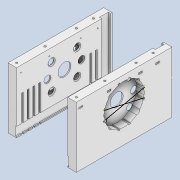
# Autodesk Inventor part: corpus_90x90x140mm_side_walls_LED_Irradiation_Firesting_ports
Saved by Autodesk Inventor 2021 (Build 250183000, 183)
## iProperties
Created: 2020-02-19
Part Number: corpus_90x90x140mm_side_walls_LED_Irradiation_Firesting_ports
Material: Acetalharz, Weiß
Document SubType Name: Modeling
Designer: Daniel
Density: 1.425 g/cm^3
Appearance: Glatt - Weiß
Author: Daniel
Autodesk Inventor part; units mm, degrees
(part 1 of 2)
ref_plane "YZ Plane" through (0, 0, 0) normal (1, 0, 0) x (0, 1, 0)
ref_plane "XZ Plane" through (0, 0, 0) normal (0, 1, 0) x (-1, 0, 0)
sketch "Skizze1" plane through (0, 0, 0) normal (0, 0, 1) x (1, 0, 0)
  line L0 (-60, 61) -> (60, 61)
  line L1 (60, 61) -> (60, -61)
  line L2 (60, -61) -> (-60, -61)
  line L3 (-60, -61) -> (-60, 61)
  line L4 (-60, 61) -> (60, -61) construction
  line L5 (60, 61) -> (-60, -61) construction
  line L6 (-45, 45.75) -> (45, 45.75)
  line L7 (45, 45.75) -> (45, -45.75)
  line L8 (45, -45.75) -> (-45, -45.75)
  line L9 (-45, -45.75) -> (-45, 45.75)
  line L10 (-45, 45.75) -> (45, -45.75) construction
  line L11 (45, 45.75) -> (-45, -45.75) construction
  line L12 (-45, -45.75) -> (-45, -61)
  line L13 (-45, -61) -> (45, -61)
  line L14 (45, -61) -> (45, -45.75)
  line L15 (45, -45.75) -> (-45, -45.75)
  line L16 (45, -43.5) -> (47, -43.5)
  line L17 (47, -43.5) -> (47, -59)
  line L18 (47, -59) -> (45, -59)
  line L19 (45, -59) -> (45, -43.5)
  line L20 (-45, -43.5) -> (-47, -43.5)
  line L21 (-47, -43.5) -> (-47, -59)
  line L22 (-47, -59) -> (-45, -59)
  line L23 (-45, -59) -> (-45, -43.5)
  point P0 (0, 0)
  dimension "d0" = 120
  dimension "d1" = 122
  dimension "d2" = 90
  dimension "d3" = 15.5
  dimension "d4" = 15.5
  dimension "d5" = 2
  dimension "d6" = 2
  dimension "d7" = 2
  dimension "d93" = 94
  dimension "d96" = 2
  constraints: 48 end point, 10 parallel, 9 point on line, 6 perpendicular, 4 midpoint, 2 horizontal
  measures "d0" distance of L0.start L0.end
  measures "d1" distance of L0.end L1.end
  measures "d2" distance of L6.start L6.end
  measures "d3" distance of L16.end L17.end
  measures "d4" distance of L20.end L21.end
  measures "d5" distance of L17.end L18.end
  measures "d6" distance of L21.end L22.end
  measures "d7" distance between parallel lines of L2 L18
  measures "d93" distance between parallel lines of L17 L21
  measures "d96" distance between parallel lines of L2 L22
extrude "Extrusion1" add sketch "Skizze1" along normal blind 168 contours L0 L1 L2 L14 L18 L17 L16 L7 L6 L9 L20 L21 L22 L12 L3
sketch "Skizze2" plane through (-60, -61, 0) normal (0, -1, 0) x (1, 0, 0)
  line L0 (10.8, 18.5) -> (109.2, 18.5)
  line L1 (109.2, 18.5) -> (109.2, 3)
  line L2 (109.2, 3) -> (10.8, 3)
  line L3 (10.8, 3) -> (10.8, 18.5)
  line L4 (10.8, 18.5) -> (109.2, 3) construction
  line L5 (109.2, 18.5) -> (10.8, 3) construction
  line L6 (105, 0) -> (120, 0) projected
  point P0 (60, 0)
  point P1 (60, 10.75)
  dimension "d10" = 10.75
  dimension "d11" = 98.4
  dimension "d12" = 15.5
  constraints: 12 end point, 2 midpoint, 2 parallel, 1 horizontal, 1 perpendicular
  measures "d10" distance of point (60, 0) point (60, 10.75)
  measures "d11" distance of L0.start L0.end
  measures "d12" distance of L0.end L1.end
extrude "Extrusion2" cut sketch "Skizze2" against normal blind 112
sketch "Skizze3" plane through (-45, 45.75, 168) normal (0, -1, 0) x (1, 0, 0)
  line L0 (-15, -168) -> (-15, 0) projected
  line L1 (105, -168) -> (105, 0) projected
  line L2 (-15, 0) -> (105, 0)
  line L3 (105, 0) -> (105, -120)
  line L4 (105, -120) -> (-15, -120)
  line L5 (-15, -120) -> (-15, 0)
  line L6 (105, 0) -> (-15, 0) construction
  line L7 (-15, 0) -> (105, -120) construction
  line L8 (105, -168) -> (105, 0) construction
  line L9 (105, 0) -> (-15, -120) construction
  circle A0 centre (45, -60) radius 45
  point P0 (45, -168)
  dimension "d16" = 120
  dimension "d17" = 90
  constraints: 12 end point, 2 parallel, 1 centre point, 1 coincident, 1 horizontal, 1 midpoint, 1 perpendicular, 1 point on line
  measures "d16" distance from line of L4 L1.end
  measures "d17" diameter of A0
extrude "Extrusion3" cut sketch "Skizze3" against normal up to surface (15.25 mm away) contours A0
sketch "Skizze4" plane through (-60, 61, 0) normal (0, 1, 0) x (1, 0, 0)
  arc A0 (105, -108) -> (15, -108) centre (60, -108) ccw projected
  circle A1 centre (60, -108) radius 45
  line L0 (120, 0) -> (120, -168) construction
  line L1 (0, 0) -> (0, -168) construction
  line L2 (120, -168) -> (0, -168) construction
  line L3 (0, -168) -> (0, -48) construction
  line L4 (0, -48) -> (120, -48) construction
  line L5 (120, -48) -> (120, -168) construction
  line L6 (0, -168) -> (120, -48) construction
  line L7 (120, -168) -> (0, -48) construction
  line L8 (24.9924, -114.4218) -> (23.5782, -113.0076)
  line L9 (23.5782, -113.0076) -> (95.0076, -41.5782)
  line L10 (95.0076, -41.5782) -> (96.4218, -42.9924)
  line L11 (96.4218, -42.9924) -> (24.9924, -114.4218)
  line L12 (59, -57.4918) -> (61, -158.5082) construction
  line L13 (61, -57.4918) -> (59, -158.5082) construction
  line L14 (23.1391, -39.7249) -> (98.2751, -114.8609)
  line L15 (98.2751, -114.8609) -> (96.8609, -116.2751)
  line L16 (96.8609, -116.2751) -> (21.7249, -41.1391)
  line L17 (21.7249, -41.1391) -> (23.1391, -39.7249)
  line L18 (113.1292, -109) -> (6.8708, -107) construction
  line L19 (6.8708, -109) -> (113.1292, -107) construction
  line L20 (30.2102, -32.6538) -> (105.3462, -107.7898)
  line L21 (103.932, -109.2041) -> (28.7959, -34.068)
  line L22 (28.7959, -34.068) -> (30.2102, -32.6538)
  line L23 (105.3462, -107.7898) -> (103.932, -109.2041)
  line L24 (37.2812, -25.5827) -> (112.4173, -100.7188)
  line L25 (111.003, -102.133) -> (35.867, -26.997)
  line L26 (35.867, -26.997) -> (37.2812, -25.5827)
  line L27 (112.4173, -100.7188) -> (111.003, -102.133)
  line L28 (44.3523, -18.5117) -> (119.4883, -93.6477)
  line L29 (118.0741, -95.0619) -> (42.9381, -19.9259)
  line L30 (42.9381, -19.9259) -> (44.3523, -18.5117)
  line L31 (119.4883, -93.6477) -> (118.0741, -95.0619)
  line L32 (51.4234, -11.4406) -> (126.5594, -86.5766)
  line L33 (125.1452, -87.9909) -> (50.0091, -12.8548)
  line L34 (50.0091, -12.8548) -> (51.4234, -11.4406)
  line L35 (126.5594, -86.5766) -> (125.1452, -87.9909)
  line L36 (16.068, -46.7959) -> (91.2041, -121.932)
  line L37 (89.7898, -123.3462) -> (14.6538, -48.2102)
  line L38 (14.6538, -48.2102) -> (16.068, -46.7959)
  line L39 (91.2041, -121.932) -> (89.7898, -123.3462)
  line L40 (23.1391, -39.7249) -> (98.2751, -114.8609)
  line L41 (96.8609, -116.2751) -> (21.7249, -41.1391)
  line L42 (21.7249, -41.1391) -> (23.1391, -39.7249)
  line L43 (98.2751, -114.8609) -> (96.8609, -116.2751)
  line L44 (30.2102, -32.6538) -> (105.3462, -107.7898)
  line L45 (103.932, -109.2041) -> (28.7959, -34.068)
  line L46 (28.7959, -34.068) -> (30.2102, -32.6538)
  line L47 (105.3462, -107.7898) -> (103.932, -109.2041)
  line L48 (37.2812, -25.5827) -> (112.4173, -100.7188)
  line L49 (111.003, -102.133) -> (35.867, -26.997)
  line L50 (35.867, -26.997) -> (37.2812, -25.5827)
  line L51 (112.4173, -100.7188) -> (111.003, -102.133)
  line L52 (44.3523, -18.5117) -> (119.4883, -93.6477)
  line L53 (118.0741, -95.0619) -> (42.9381, -19.9259)
  line L54 (42.9381, -19.9259) -> (44.3523, -18.5117)
  line L55 (119.4883, -93.6477) -> (118.0741, -95.0619)
  line L56 (8.997, -53.867) -> (84.133, -129.003)
  line L57 (82.7188, -130.4173) -> (7.5827, -55.2812)
  line L58 (7.5827, -55.2812) -> (8.997, -53.867)
  line L59 (84.133, -129.003) -> (82.7188, -130.4173)
  line L60 (16.068, -46.7959) -> (91.2041, -121.932)
  line L61 (89.7898, -123.3462) -> (14.6538, -48.2102)
  line L62 (14.6538, -48.2102) -> (16.068, -46.7959)
  line L63 (91.2041, -121.932) -> (89.7898, -123.3462)
  line L64 (23.1391, -39.7249) -> (98.2751, -114.8609)
  line L65 (96.8609, -116.2751) -> (21.7249, -41.1391)
  line L66 (21.7249, -41.1391) -> (23.1391, -39.7249)
  line L67 (98.2751, -114.8609) -> (96.8609, -116.2751)
  line L68 (30.2102, -32.6538) -> (105.3462, -107.7898)
  line L69 (103.932, -109.2041) -> (28.7959, -34.068)
  line L70 (28.7959, -34.068) -> (30.2102, -32.6538)
  line L71 (105.3462, -107.7898) -> (103.932, -109.2041)
  line L72 (37.2812, -25.5827) -> (112.4173, -100.7188)
  line L73 (111.003, -102.133) -> (35.867, -26.997)
  line L74 (35.867, -26.997) -> (37.2812, -25.5827)
  line L75 (112.4173, -100.7188) -> (111.003, -102.133)
  line L76 (1.9259, -60.9381) -> (77.0619, -136.0741)
  line L77 (75.6477, -137.4883) -> (0.5117, -62.3523)
  line L78 (0.5117, -62.3523) -> (1.9259, -60.9381)
  line L79 (77.0619, -136.0741) -> (75.6477, -137.4883)
  line L80 (8.997, -53.867) -> (84.133, -129.003)
  line L81 (82.7188, -130.4173) -> (7.5827, -55.2812)
  line L82 (7.5827, -55.2812) -> (8.997, -53.867)
  line L83 (84.133, -129.003) -> (82.7188, -130.4173)
  line L84 (16.068, -46.7959) -> (91.2041, -121.932)
  line L85 (89.7898, -123.3462) -> (14.6538, -48.2102)
  line L86 (14.6538, -48.2102) -> (16.068, -46.7959)
  line L87 (91.2041, -121.932) -> (89.7898, -123.3462)
  line L88 (23.1391, -39.7249) -> (98.2751, -114.8609)
  line L89 (96.8609, -116.2751) -> (21.7249, -41.1391)
  line L90 (21.7249, -41.1391) -> (23.1391, -39.7249)
  line L91 (98.2751, -114.8609) -> (96.8609, -116.2751)
  line L92 (30.2102, -32.6538) -> (105.3462, -107.7898)
  line L93 (103.932, -109.2041) -> (28.7959, -34.068)
  line L94 (28.7959, -34.068) -> (30.2102, -32.6538)
  line L95 (105.3462, -107.7898) -> (103.932, -109.2041)
  line L96 (-5.1452, -68.0091) -> (69.9909, -143.1452)
  line L97 (68.5766, -144.5594) -> (-6.5594, -69.4234)
  line L98 (-6.5594, -69.4234) -> (-5.1452, -68.0091)
  line L99 (69.9909, -143.1452) -> (68.5766, -144.5594)
  line L100 (1.9259, -60.9381) -> (77.0619, -136.0741)
  line L101 (75.6477, -137.4883) -> (0.5117, -62.3523)
  line L102 (0.5117, -62.3523) -> (1.9259, -60.9381)
  line L103 (77.0619, -136.0741) -> (75.6477, -137.4883)
  line L104 (8.997, -53.867) -> (84.133, -129.003)
  line L105 (82.7188, -130.4173) -> (7.5827, -55.2812)
  line L106 (7.5827, -55.2812) -> (8.997, -53.867)
  line L107 (84.133, -129.003) -> (82.7188, -130.4173)
  line L108 (16.068, -46.7959) -> (91.2041, -121.932)
  line L109 (89.7898, -123.3462) -> (14.6538, -48.2102)
  line L110 (14.6538, -48.2102) -> (16.068, -46.7959)
  line L111 (91.2041, -121.932) -> (89.7898, -123.3462)
  line L112 (23.1391, -39.7249) -> (98.2751, -114.8609)
  line L113 (96.8609, -116.2751) -> (21.7249, -41.1391)
  line L114 (21.7249, -41.1391) -> (23.1391, -39.7249)
  line L115 (98.2751, -114.8609) -> (96.8609, -116.2751)
  line L116 (16.5071, -105.9365) -> (87.9365, -34.5071)
  line L117 (89.3507, -35.9213) -> (17.9213, -107.3507)
  line L118 (17.9213, -107.3507) -> (16.5071, -105.9365)
  line L119 (87.9365, -34.5071) -> (89.3507, -35.9213)
  line L120 (9.4361, -98.8655) -> (80.8655, -27.4361)
  line L121 (82.2797, -28.8503) -> (10.8503, -100.2797)
  line L122 (10.8503, -100.2797) -> (9.4361, -98.8655)
  line L123 (80.8655, -27.4361) -> (82.2797, -28.8503)
  line L124 (2.365, -91.7944) -> (73.7944, -20.365)
  line L125 (75.2086, -21.7792) -> (3.7792, -93.2086)
  line L126 (3.7792, -93.2086) -> (2.365, -91.7944)
  line L127 (73.7944, -20.365) -> (75.2086, -21.7792)
  line L128 (-4.7061, -84.7233) -> (66.7233, -13.2939)
  line L129 (68.1375, -14.7081) -> (-3.2919, -86.1375)
  line L130 (-3.2919, -86.1375) -> (-4.7061, -84.7233)
  line L131 (66.7233, -13.2939) -> (68.1375, -14.7081)
  line L132 (30.6493, -120.0787) -> (102.0787, -48.6493)
  line L133 (103.4929, -50.0635) -> (32.0635, -121.4929)
  line L134 (32.0635, -121.4929) -> (30.6493, -120.0787)
  line L135 (102.0787, -48.6493) -> (103.4929, -50.0635)
  line L136 (23.5782, -113.0076) -> (95.0076, -41.5782)
  line L137 (96.4218, -42.9924) -> (24.9924, -114.4218)
  line L138 (24.9924, -114.4218) -> (23.5782, -113.0076)
  line L139 (95.0076, -41.5782) -> (96.4218, -42.9924)
  line L140 (16.5071, -105.9365) -> (87.9365, -34.5071)
  line L141 (89.3507, -35.9213) -> (17.9213, -107.3507)
  line L142 (17.9213, -107.3507) -> (16.5071, -105.9365)
  line L143 (87.9365, -34.5071) -> (89.3507, -35.9213)
  line L144 (9.4361, -98.8655) -> (80.8655, -27.4361)
  line L145 (82.2797, -28.8503) -> (10.8503, -100.2797)
  line L146 (10.8503, -100.2797) -> (9.4361, -98.8655)
  line L147 (80.8655, -27.4361) -> (82.2797, -28.8503)
  line L148 (2.365, -91.7944) -> (73.7944, -20.365)
  line L149 (75.2086, -21.7792) -> (3.7792, -93.2086)
  line L150 (3.7792, -93.2086) -> (2.365, -91.7944)
  line L151 (73.7944, -20.365) -> (75.2086, -21.7792)
  line L152 (37.7203, -127.1497) -> (109.1497, -55.7203)
  line L153 (110.5639, -57.1345) -> (39.1345, -128.5639)
  line L154 (39.1345, -128.5639) -> (37.7203, -127.1497)
  line L155 (109.1497, -55.7203) -> (110.5639, -57.1345)
  line L156 (30.6493, -120.0787) -> (102.0787, -48.6493)
  line L157 (103.4929, -50.0635) -> (32.0635, -121.4929)
  line L158 (32.0635, -121.4929) -> (30.6493, -120.0787)
  line L159 (102.0787, -48.6493) -> (103.4929, -50.0635)
  line L160 (23.5782, -113.0076) -> (95.0076, -41.5782)
  line L161 (96.4218, -42.9924) -> (24.9924, -114.4218)
  line L162 (24.9924, -114.4218) -> (23.5782, -113.0076)
  line L163 (95.0076, -41.5782) -> (96.4218, -42.9924)
  line L164 (16.5071, -105.9365) -> (87.9365, -34.5071)
  line L165 (89.3507, -35.9213) -> (17.9213, -107.3507)
  line L166 (17.9213, -107.3507) -> (16.5071, -105.9365)
  line L167 (87.9365, -34.5071) -> (89.3507, -35.9213)
  line L168 (9.4361, -98.8655) -> (80.8655, -27.4361)
  line L169 (82.2797, -28.8503) -> (10.8503, -100.2797)
  line L170 (10.8503, -100.2797) -> (9.4361, -98.8655)
  line L171 (80.8655, -27.4361) -> (82.2797, -28.8503)
  line L172 (44.7914, -134.2208) -> (116.2208, -62.7914)
  line L173 (117.635, -64.2056) -> (46.2056, -135.635)
  line L174 (46.2056, -135.635) -> (44.7914, -134.2208)
  line L175 (116.2208, -62.7914) -> (117.635, -64.2056)
  line L176 (37.7203, -127.1497) -> (109.1497, -55.7203)
  line L177 (110.5639, -57.1345) -> (39.1345, -128.5639)
  line L178 (39.1345, -128.5639) -> (37.7203, -127.1497)
  line L179 (109.1497, -55.7203) -> (110.5639, -57.1345)
  line L180 (30.6493, -120.0787) -> (102.0787, -48.6493)
  line L181 (103.4929, -50.0635) -> (32.0635, -121.4929)
  line L182 (32.0635, -121.4929) -> (30.6493, -120.0787)
  line L183 (102.0787, -48.6493) -> (103.4929, -50.0635)
  line L184 (23.5782, -113.0076) -> (95.0076, -41.5782)
  line L185 (96.4218, -42.9924) -> (24.9924, -114.4218)
  line L186 (24.9924, -114.4218) -> (23.5782, -113.0076)
  line L187 (95.0076, -41.5782) -> (96.4218, -42.9924)
  line L188 (16.5071, -105.9365) -> (87.9365, -34.5071)
  line L189 (89.3507, -35.9213) -> (17.9213, -107.3507)
  line L190 (17.9213, -107.3507) -> (16.5071, -105.9365)
  line L191 (87.9365, -34.5071) -> (89.3507, -35.9213)
  line L192 (51.8625, -141.2919) -> (123.2919, -69.8625)
  line L193 (124.7061, -71.2767) -> (53.2767, -142.7061)
  line L194 (53.2767, -142.7061) -> (51.8625, -141.2919)
  line L195 (123.2919, -69.8625) -> (124.7061, -71.2767)
  line L196 (44.7914, -134.2208) -> (116.2208, -62.7914)
  line L197 (117.635, -64.2056) -> (46.2056, -135.635)
  line L198 (46.2056, -135.635) -> (44.7914, -134.2208)
  line L199 (116.2208, -62.7914) -> (117.635, -64.2056)
  line L200 (37.7203, -127.1497) -> (109.1497, -55.7203)
  line L201 (110.5639, -57.1345) -> (39.1345, -128.5639)
  line L202 (39.1345, -128.5639) -> (37.7203, -127.1497)
  line L203 (109.1497, -55.7203) -> (110.5639, -57.1345)
  line L204 (30.6493, -120.0787) -> (102.0787, -48.6493)
  line L205 (103.4929, -50.0635) -> (32.0635, -121.4929)
  line L206 (32.0635, -121.4929) -> (30.6493, -120.0787)
  line L207 (102.0787, -48.6493) -> (103.4929, -50.0635)
  line L208 (23.5782, -113.0076) -> (95.0076, -41.5782)
  line L209 (96.4218, -42.9924) -> (24.9924, -114.4218)
  line L210 (24.9924, -114.4218) -> (23.5782, -113.0076)
  line L211 (95.0076, -41.5782) -> (96.4218, -42.9924)
  point P0 (60, 0)
  point P1 (60, -79.4142)
  point P2 (65.6569, -85.0711)
  point P3 (60, -90.7279)
  point P4 (54.3431, -85.0711)
  point P5 (58.5858, -78)
  point P6 (52.9289, -83.6569)
  point P7 (47.2721, -78)
  point P8 (52.9289, -72.3431)
  point P9 (60, -76.5858)
  point P10 (54.3431, -70.9289)
  point P11 (60, -65.2721)
  point P12 (65.6569, -70.9289)
  point P13 (61.4142, -78)
  point P14 (67.0711, -72.3431)
  point P15 (72.7279, -78)
  point P16 (67.0711, -83.6569)
  point P17 (75.5563, -63.8579)
  point P18 (81.2132, -58.201)
  point P19 (86.8701, -63.8579)
  point P20 (81.2132, -69.5147)
  point P21 (74.1421, -62.4437)
  point P22 (68.4853, -56.7868)
  point P23 (74.1421, -51.1299)
  point P24 (79.799, -56.7868)
  point P25 (88.2843, -48.3015)
  point P26 (82.6274, -42.6447)
  point P27 (81.2132, -41.2304)
  point P28 (75.8765, -35.8937)
  point P29 (45.846, -65.2839)
  point P30 (41.1745, -67.127)
  point P31 (71.7027, -34.5483)
  point P32 (72.7279, -35.5736)
  point P33 (67.0711, -41.2304)
  point P34 (61.4142, -35.5736)
  point P35 (60, -34.1594)
  point P36 (58.5858, -35.5736)
  point P37 (52.9289, -41.2304)
  point P38 (47.2721, -35.5736)
  point P39 (48.2973, -34.5483)
  point P40 (78.8255, -67.127)
  point P41 (74.154, -65.2839)
  point P42 (44.1235, -35.8937)
  point P43 (38.7868, -41.2304)
  point P44 (37.3726, -42.6447)
  point P45 (31.7157, -48.3015)
  point P46 (30.3015, -49.7157)
  point P47 (24.6447, -55.3726)
  point P48 (38.0106, -68.7385)
  point P49 (36.2324, -69.7887)
  point P50 (23.2304, -56.7868)
  point P51 (17.8937, -62.1235)
  point P52 (16.5483, -66.2973)
  point P53 (17.5736, -65.2721)
  point P54 (23.2304, -70.9289)
  point P55 (17.5736, -76.5858)
  point P56 (23.1541, -82.1663)
  point P57 (22.0215, -83.8622)
  point P58 (16.1594, -78)
  point P59 (17.5736, -79.4142)
  point P60 (23.2304, -85.0711)
  point P61 (17.5736, -90.7279)
  point P62 (18.1942, -91.3485)
  point P63 (19.127, -89.1745)
  point P64 (17.2839, -93.846)
  point P65 (17.4299, -93.4127)
  point P66 (23.2304, -99.2132)
  point P67 (24.6447, -100.6274)
  point P68 (30.3015, -106.2843)
  point P69 (31.7157, -107.6985)
  point P70 (37.3726, -113.3553)
  point P71 (38.7868, -114.7696)
  point P72 (44.1235, -120.1063)
  point P73 (48.2973, -121.4517)
  point P74 (47.2721, -120.4264)
  point P75 (52.9289, -114.7696)
  point P76 (58.5858, -120.4264)
  point P77 (96.8459, -82.1663)
  point P78 (97.9785, -83.8622)
  point P79 (60, -121.8406)
  point P80 (22.0215, -83.8622)
  point P81 (23.1541, -82.1663)
  point P82 (61.4142, -120.4264)
  point P83 (67.0711, -114.7696)
  point P84 (72.7279, -120.4264)
  point P85 (71.7027, -121.4517)
  point P86 (75.8765, -120.1063)
  point P87 (81.2132, -114.7696)
  point P88 (36.2324, -69.7887)
  point P89 (38.0106, -68.7385)
  point P90 (82.6274, -113.3553)
  point P91 (88.2843, -107.6985)
  point P92 (89.6985, -106.2843)
  point P93 (95.3553, -100.6274)
  point P94 (96.7696, -99.2132)
  point P95 (102.5701, -93.4127)
  point P96 (102.7161, -93.846)
  point P97 (100.873, -89.1745)
  point P98 (101.8058, -91.3485)
  point P99 (102.4264, -90.7279)
  point P100 (96.7696, -85.0711)
  point P101 (102.4264, -79.4142)
  point P102 (103.8406, -78)
  point P103 (97.9785, -83.8622)
  point P104 (96.8459, -82.1663)
  point P105 (102.4264, -76.5858)
  point P106 (96.7696, -70.9289)
  point P107 (102.4264, -65.2721)
  point P108 (103.4517, -66.2973)
  point P109 (102.1063, -62.1235)
  point P110 (96.7696, -56.7868)
  point P111 (95.3553, -55.3726)
  point P112 (89.6985, -49.7157)
  point P113 (52.9289, -86.4853)
  point P114 (58.5858, -92.1421)
  point P115 (52.9289, -97.799)
  point P116 (47.2721, -92.1421)
  point P117 (51.5147, -85.0711)
  point P118 (45.8579, -90.7279)
  point P119 (40.201, -85.0711)
  point P120 (45.8579, -79.4142)
  point P121 (45.8579, -93.5563)
  point P122 (51.5147, -99.2132)
  point P123 (45.8579, -104.8701)
  point P124 (40.201, -99.2132)
  point P125 (37.3726, -99.2132)
  point P126 (31.7157, -104.8701)
  point P127 (26.0589, -99.2132)
  point P128 (31.7157, -93.5563)
  point P129 (72.7279, -49.7157)
  point P130 (67.0711, -55.3726)
  point P131 (61.4142, -49.7157)
  point P132 (67.0711, -44.0589)
  point P133 (58.5858, -63.8579)
  point P134 (52.9289, -69.5147)
  point P135 (47.2721, -63.8579)
  point P136 (52.9289, -58.201)
  point P137 (44.4437, -78)
  point P138 (38.7868, -83.6569)
  point P139 (33.1299, -78)
  point P140 (38.7868, -72.3431)
  point P141 (37.3726, -85.0711)
  point P142 (31.7157, -90.7279)
  point P143 (26.0589, -85.0711)
  point P144 (31.7157, -79.4142)
  point P145 (30.3015, -92.1421)
  point P146 (24.6447, -97.799)
  point P147 (18.9878, -92.1421)
  point P148 (24.6447, -86.4853)
  point P149 (65.6569, -42.6447)
  point P150 (60, -48.3015)
  point P151 (54.3431, -42.6447)
  point P152 (60, -36.9878)
  point P153 (51.5147, -56.7868)
  point P154 (45.8579, -62.4437)
  point P155 (40.201, -56.7868)
  point P156 (45.8579, -51.1299)
  point P157 (37.3726, -70.9289)
  point P158 (31.7157, -76.5858)
  point P159 (26.0589, -70.9289)
  point P160 (31.7157, -65.2721)
  point P161 (30.3015, -78)
  point P162 (24.6447, -83.6569)
  point P163 (18.9878, -78)
  point P164 (24.6447, -72.3431)
  point P165 (37.3726, -56.7868)
  point P166 (31.7157, -62.4437)
  point P167 (26.0589, -56.7868)
  point P168 (31.7157, -51.1299)
  point P169 (30.3015, -63.8579)
  point P170 (24.6447, -69.5147)
  point P171 (18.9878, -63.8579)
  point P172 (24.6447, -58.201)
  point P173 (44.4437, -49.7157)
  point P174 (38.7868, -55.3726)
  point P175 (33.1299, -49.7157)
  point P176 (38.7868, -44.0589)
  point P177 (51.5147, -42.6447)
  point P178 (45.8579, -48.3015)
  point P179 (40.201, -42.6447)
  point P180 (45.8579, -36.9878)
  point P181 (44.4437, -63.8579)
  point P182 (38.7868, -69.5147)
  point P183 (33.1299, -63.8579)
  point P184 (38.7868, -58.201)
  point P185 (58.5858, -49.7157)
  point P186 (52.9289, -55.3726)
  point P187 (47.2721, -49.7157)
  point P188 (52.9289, -44.0589)
  point P189 (51.5147, -70.9289)
  point P190 (45.8579, -76.5858)
  point P191 (40.201, -70.9289)
  point P192 (45.8579, -65.2721)
  point P193 (65.6569, -56.7868)
  point P194 (60, -62.4437)
  point P195 (54.3431, -56.7868)
  point P196 (60, -51.1299)
  point P197 (79.799, -42.6447)
  point P198 (74.1421, -48.3015)
  point P199 (68.4853, -42.6447)
  dimension "d20" = 120
  dimension "d21" = 2
  dimension "d22" = 2
  dimension "d25" = 10
  dimension "d28" = 10
  dimension "d33" = 10
  dimension "d36" = 10
  constraints: 416 end point, 8 perpendicular, 6 parallel, 4 midpoint, 2 point on line, 1 centre point, 1 coincident, 1 horizontal, 390 other
  measures "d20" distance between parallel lines of L2 L4
  measures "d21" distance of L9.end L10.end
  measures "d22" distance of L14.end L15.end
  measures "d25" distance of L14.start L20.start
  measures "d28" distance of L14.start L38.end
  measures "d33" distance of L8.end L116.start
  measures "d36" distance of L8.end L132.start
extrude "Extrusion4" [suppressed]
sketch "Skizze5" plane through (-60, 61, 0) normal (0, 1, 0) x (1, 0, 0)
  line L0 (120, 0) -> (120, -168) construction
  line L1 (0, 0) -> (0, -168) construction
  line L2 (120, -168) -> (0, -168) construction
  line L3 (0, -168) -> (0, -48) construction
  line L4 (0, -48) -> (120, -48) construction
  line L5 (120, -48) -> (120, -168) construction
  line L6 (105, -168) -> (120, -168) construction
  line L7 (120, -168) -> (0, -48) construction
  line L8 (0, -168) -> (15, -168) construction
  line L9 (0, -168) -> (120, -48) construction
  line L10 (112.5, -160.5) -> (7.5, -160.5) construction
  line L11 (7.5, -160.5) -> (7.5, -55.5) construction
  line L12 (7.5, -55.5) -> (112.5, -55.5) construction
  line L13 (112.5, -55.5) -> (112.5, -160.5) construction
  line L14 (112.5, -160.5) -> (7.5, -55.5) construction
  line L15 (7.5, -160.5) -> (112.5, -55.5) construction
  circle A0 centre (112.5, -160.5) radius 1.35
  circle A1 centre (7.5, -160.5) radius 1.35
  circle A2 centre (7.5, -55.5) radius 1.35
  circle A3 centre (112.5, -55.5) radius 1.35
  point P0 (60, 0)
  point P1 (60, -108)
  dimension "d41" = 120
  dimension "d42" = 2.7
  dimension "d43" = 2.7
  dimension "d44" = 2.7
  dimension "d45" = 2.7
  dimension "d46" = 105
  constraints: 24 end point, 4 centre point, 4 coincident, 4 parallel, 3 midpoint, 2 horizontal, 2 perpendicular, 2 point on line
  measures "d41" distance between parallel lines of L2 L4
  measures "d42" diameter of A0
  measures "d43" diameter of A1
  measures "d44" diameter of A2
  measures "d45" diameter of A3
  measures "d46" distance of L10.start L10.end
extrude "Extrusion5" cut sketch "Skizze5" against normal blind 30
sketch "Skizze7" plane through (-60, -61, 0) normal (0, -1, 0) x (1, 0, 0)
  line L0 (0, 0) -> (0, 168) construction
  line L1 (120, 0) -> (120, 168) construction
  line L2 (0, 168) -> (120, 168) construction
  line L3 (120, 168) -> (120, 48) construction
  line L4 (0, 48) -> (0, 168) construction
  line L5 (0, 168) -> (15, 168) construction
  line L6 (105, 168) -> (120, 168) construction
  line L7 (-105.8605, 110.8419) -> (-11.8605, 110.8419)
  line L8 (-11.8605, 110.8419) -> (-11.8605, 107.8419)
  line L9 (-11.8605, 107.8419) -> (-105.8605, 107.8419)
  line L10 (-105.8605, 107.8419) -> (-105.8605, 110.8419)
  line L11 (-58.8605, 109.3419) -> (-58.8605, 19.8419) construction
  line L12 (120, 168) -> (0, 168) construction
  line L13 (107, 129.5) -> (107, 126.5)
  line L14 (13, 129.5) -> (107, 129.5)
  line L15 (107, 126.5) -> (13, 126.5)
  line L16 (13, 126.5) -> (13, 129.5)
  line L17 (107, 139.5) -> (107, 136.5)
  line L18 (13, 139.5) -> (107, 139.5)
  line L19 (107, 136.5) -> (13, 136.5)
  line L20 (13, 136.5) -> (13, 139.5)
  line L21 (107, 149.5) -> (107, 146.5)
  line L22 (13, 149.5) -> (107, 149.5)
  line L23 (107, 146.5) -> (13, 146.5)
  line L24 (13, 146.5) -> (13, 149.5)
  line L25 (107, 159.5) -> (107, 156.5)
  line L26 (13, 159.5) -> (107, 159.5)
  line L27 (107, 156.5) -> (13, 156.5)
  line L28 (13, 156.5) -> (13, 159.5)
  line L29 (-11.8605, 100.8419) -> (-11.8605, 97.8419)
  line L30 (-105.8605, 100.8419) -> (-11.8605, 100.8419)
  line L31 (-11.8605, 97.8419) -> (-105.8605, 97.8419)
  line L32 (-105.8605, 97.8419) -> (-105.8605, 100.8419)
  line L33 (-11.8605, 110.8419) -> (-11.8605, 107.8419)
  line L34 (-105.8605, 110.8419) -> (-11.8605, 110.8419)
  line L35 (-11.8605, 107.8419) -> (-105.8605, 107.8419)
  line L36 (-105.8605, 107.8419) -> (-105.8605, 110.8419)
  line L37 (107, 129.5) -> (107, 126.5)
  line L38 (13, 129.5) -> (107, 129.5)
  line L39 (107, 126.5) -> (13, 126.5)
  line L40 (13, 126.5) -> (13, 129.5)
  line L41 (107, 139.5) -> (107, 136.5)
  line L42 (13, 139.5) -> (107, 139.5)
  line L43 (107, 136.5) -> (13, 136.5)
  line L44 (13, 136.5) -> (13, 139.5)
  line L45 (107, 149.5) -> (107, 146.5)
  line L46 (13, 149.5) -> (107, 149.5)
  line L47 (107, 146.5) -> (13, 146.5)
  line L48 (13, 146.5) -> (13, 149.5)
  line L49 (-11.8605, 90.8419) -> (-11.8605, 87.8419)
  line L50 (-105.8605, 90.8419) -> (-11.8605, 90.8419)
  line L51 (-11.8605, 87.8419) -> (-105.8605, 87.8419)
  line L52 (-105.8605, 87.8419) -> (-105.8605, 90.8419)
  line L53 (-11.8605, 100.8419) -> (-11.8605, 97.8419)
  line L54 (-105.8605, 100.8419) -> (-11.8605, 100.8419)
  line L55 (-11.8605, 97.8419) -> (-105.8605, 97.8419)
  line L56 (-105.8605, 97.8419) -> (-105.8605, 100.8419)
  line L57 (-11.8605, 110.8419) -> (-11.8605, 107.8419)
  line L58 (-105.8605, 110.8419) -> (-11.8605, 110.8419)
  line L59 (-11.8605, 107.8419) -> (-105.8605, 107.8419)
  line L60 (-105.8605, 107.8419) -> (-105.8605, 110.8419)
  line L61 (107, 129.5) -> (107, 126.5)
  line L62 (13, 129.5) -> (107, 129.5)
  line L63 (107, 126.5) -> (13, 126.5)
  line L64 (13, 126.5) -> (13, 129.5)
  line L65 (107, 139.5) -> (107, 136.5)
  line L66 (13, 139.5) -> (107, 139.5)
  line L67 (107, 136.5) -> (13, 136.5)
  line L68 (13, 136.5) -> (13, 139.5)
  line L69 (-11.8605, 80.8419) -> (-11.8605, 77.8419)
  line L70 (-105.8605, 80.8419) -> (-11.8605, 80.8419)
  line L71 (-11.8605, 77.8419) -> (-105.8605, 77.8419)
  line L72 (-105.8605, 77.8419) -> (-105.8605, 80.8419)
  line L73 (-11.8605, 90.8419) -> (-11.8605, 87.8419)
  line L74 (-105.8605, 90.8419) -> (-11.8605, 90.8419)
  line L75 (-11.8605, 87.8419) -> (-105.8605, 87.8419)
  line L76 (-105.8605, 87.8419) -> (-105.8605, 90.8419)
  line L77 (-11.8605, 100.8419) -> (-11.8605, 97.8419)
  line L78 (-105.8605, 100.8419) -> (-11.8605, 100.8419)
  line L79 (-11.8605, 97.8419) -> (-105.8605, 97.8419)
  line L80 (-105.8605, 97.8419) -> (-105.8605, 100.8419)
  line L81 (-11.8605, 110.8419) -> (-11.8605, 107.8419)
  line L82 (-105.8605, 110.8419) -> (-11.8605, 110.8419)
  line L83 (-11.8605, 107.8419) -> (-105.8605, 107.8419)
  line L84 (-105.8605, 107.8419) -> (-105.8605, 110.8419)
  line L85 (107, 129.5) -> (107, 126.5)
  line L86 (13, 129.5) -> (107, 129.5)
  line L87 (107, 126.5) -> (13, 126.5)
  line L88 (13, 126.5) -> (13, 129.5)
  line L89 (-11.8605, 70.8419) -> (-11.8605, 67.8419)
  line L90 (-105.8605, 70.8419) -> (-11.8605, 70.8419)
  line L91 (-11.8605, 67.8419) -> (-105.8605, 67.8419)
  line L92 (-105.8605, 67.8419) -> (-105.8605, 70.8419)
  line L93 (-11.8605, 80.8419) -> (-11.8605, 77.8419)
  line L94 (-105.8605, 80.8419) -> (-11.8605, 80.8419)
  line L95 (-11.8605, 77.8419) -> (-105.8605, 77.8419)
  line L96 (-105.8605, 77.8419) -> (-105.8605, 80.8419)
  line L97 (-11.8605, 90.8419) -> (-11.8605, 87.8419)
  line L98 (-105.8605, 90.8419) -> (-11.8605, 90.8419)
  line L99 (-11.8605, 87.8419) -> (-105.8605, 87.8419)
  line L100 (-105.8605, 87.8419) -> (-105.8605, 90.8419)
  line L101 (-11.8605, 100.8419) -> (-11.8605, 97.8419)
  line L102 (-105.8605, 100.8419) -> (-11.8605, 100.8419)
  line L103 (-11.8605, 97.8419) -> (-105.8605, 97.8419)
  line L104 (-105.8605, 97.8419) -> (-105.8605, 100.8419)
  line L105 (-11.8605, 110.8419) -> (-11.8605, 107.8419)
  line L106 (-105.8605, 110.8419) -> (-11.8605, 110.8419)
  line L107 (-11.8605, 107.8419) -> (-105.8605, 107.8419)
  line L108 (-105.8605, 107.8419) -> (-105.8605, 110.8419)
  line L109 (-11.8605, 60.8419) -> (-11.8605, 57.8419)
  line L110 (-105.8605, 60.8419) -> (-11.8605, 60.8419)
  line L111 (-11.8605, 57.8419) -> (-105.8605, 57.8419)
  line L112 (-105.8605, 57.8419) -> (-105.8605, 60.8419)
  line L113 (-11.8605, 70.8419) -> (-11.8605, 67.8419)
  line L114 (-105.8605, 70.8419) -> (-11.8605, 70.8419)
  line L115 (-11.8605, 67.8419) -> (-105.8605, 67.8419)
  line L116 (-105.8605, 67.8419) -> (-105.8605, 70.8419)
  line L117 (-11.8605, 80.8419) -> (-11.8605, 77.8419)
  line L118 (-105.8605, 80.8419) -> (-11.8605, 80.8419)
  line L119 (-11.8605, 77.8419) -> (-105.8605, 77.8419)
  line L120 (-105.8605, 77.8419) -> (-105.8605, 80.8419)
  line L121 (-11.8605, 90.8419) -> (-11.8605, 87.8419)
  line L122 (-105.8605, 90.8419) -> (-11.8605, 90.8419)
  line L123 (-11.8605, 87.8419) -> (-105.8605, 87.8419)
  line L124 (-105.8605, 87.8419) -> (-105.8605, 90.8419)
  line L125 (-11.8605, 100.8419) -> (-11.8605, 97.8419)
  line L126 (-105.8605, 100.8419) -> (-11.8605, 100.8419)
  line L127 (-11.8605, 97.8419) -> (-105.8605, 97.8419)
  line L128 (-105.8605, 97.8419) -> (-105.8605, 100.8419)
  line L129 (107, 99.5) -> (107, 96.5)
  line L130 (13, 99.5) -> (107, 99.5)
  line L131 (107, 96.5) -> (13, 96.5)
  line L132 (13, 96.5) -> (13, 99.5)
  line L133 (107, 109.5) -> (107, 106.5)
  line L134 (13, 109.5) -> (107, 109.5)
  line L135 (107, 106.5) -> (13, 106.5)
  line L136 (13, 106.5) -> (13, 109.5)
  line L137 (107, 119.5) -> (107, 116.5)
  line L138 (13, 119.5) -> (107, 119.5)
  line L139 (107, 116.5) -> (13, 116.5)
  line L140 (13, 116.5) -> (13, 119.5)
  line L141 (107, 129.5) -> (107, 126.5)
  line L142 (13, 129.5) -> (107, 129.5)
  line L143 (107, 126.5) -> (13, 126.5)
  line L144 (13, 126.5) -> (13, 129.5)
  line L145 (107, 99.5) -> (107, 96.5)
  line L146 (13, 99.5) -> (107, 99.5)
  line L147 (107, 96.5) -> (13, 96.5)
  line L148 (13, 96.5) -> (13, 99.5)
  line L149 (107, 109.5) -> (107, 106.5)
  line L150 (13, 109.5) -> (107, 109.5)
  line L151 (107, 106.5) -> (13, 106.5)
  line L152 (13, 106.5) -> (13, 109.5)
  line L153 (107, 119.5) -> (107, 116.5)
  line L154 (13, 119.5) -> (107, 119.5)
  line L155 (107, 116.5) -> (13, 116.5)
  line L156 (13, 116.5) -> (13, 119.5)
  line L157 (107, 99.5) -> (107, 96.5)
  line L158 (13, 99.5) -> (107, 99.5)
  line L159 (107, 96.5) -> (13, 96.5)
  line L160 (13, 96.5) -> (13, 99.5)
  line L161 (107, 109.5) -> (107, 106.5)
  line L162 (13, 109.5) -> (107, 109.5)
  line L163 (107, 106.5) -> (13, 106.5)
  line L164 (13, 106.5) -> (13, 109.5)
  line L165 (107, 99.5) -> (107, 96.5)
  line L166 (13, 99.5) -> (107, 99.5)
  line L167 (107, 96.5) -> (13, 96.5)
  line L168 (13, 96.5) -> (13, 99.5)
  line L169 (107, 69.5) -> (107, 66.5)
  line L170 (13, 69.5) -> (107, 69.5)
  line L171 (107, 66.5) -> (13, 66.5)
  line L172 (13, 66.5) -> (13, 69.5)
  line L173 (107, 79.5) -> (107, 76.5)
  line L174 (13, 79.5) -> (107, 79.5)
  line L175 (107, 76.5) -> (13, 76.5)
  line L176 (13, 76.5) -> (13, 79.5)
  line L177 (107, 89.5) -> (107, 86.5)
  line L178 (13, 89.5) -> (107, 89.5)
  line L179 (107, 86.5) -> (13, 86.5)
  line L180 (13, 86.5) -> (13, 89.5)
  line L181 (107, 99.5) -> (107, 96.5)
  line L182 (13, 99.5) -> (107, 99.5)
  line L183 (107, 96.5) -> (13, 96.5)
  line L184 (13, 96.5) -> (13, 99.5)
  line L185 (107, 69.5) -> (107, 66.5)
  line L186 (13, 69.5) -> (107, 69.5)
  line L187 (107, 66.5) -> (13, 66.5)
  line L188 (13, 66.5) -> (13, 69.5)
  line L189 (107, 79.5) -> (107, 76.5)
  line L190 (13, 79.5) -> (107, 79.5)
  line L191 (107, 76.5) -> (13, 76.5)
  line L192 (13, 76.5) -> (13, 79.5)
  line L193 (107, 89.5) -> (107, 86.5)
  line L194 (13, 89.5) -> (107, 89.5)
  line L195 (107, 86.5) -> (13, 86.5)
  line L196 (13, 86.5) -> (13, 89.5)
  line L197 (107, 69.5) -> (107, 66.5)
  line L198 (13, 69.5) -> (107, 69.5)
  line L199 (107, 66.5) -> (13, 66.5)
  line L200 (13, 66.5) -> (13, 69.5)
  line L201 (107, 79.5) -> (107, 76.5)
  line L202 (13, 79.5) -> (107, 79.5)
  line L203 (107, 76.5) -> (13, 76.5)
  line L204 (13, 76.5) -> (13, 79.5)
  line L205 (107, 69.5) -> (107, 66.5)
  line L206 (13, 69.5) -> (107, 69.5)
  line L207 (107, 66.5) -> (13, 66.5)
  line L208 (13, 66.5) -> (13, 69.5)
  line L209 (107, 39.5) -> (107, 36.5)
  line L210 (13, 39.5) -> (107, 39.5)
  line L211 (107, 36.5) -> (13, 36.5)
  line L212 (13, 36.5) -> (13, 39.5)
  line L213 (107, 49.5) -> (107, 46.5)
  line L214 (13, 49.5) -> (107, 49.5)
  line L215 (107, 46.5) -> (13, 46.5)
  line L216 (13, 46.5) -> (13, 49.5)
  line L217 (107, 59.5) -> (107, 56.5)
  line L218 (13, 59.5) -> (107, 59.5)
  line L219 (107, 56.5) -> (13, 56.5)
  line L220 (13, 56.5) -> (13, 59.5)
  line L221 (107, 69.5) -> (107, 66.5)
  line L222 (13, 69.5) -> (107, 69.5)
  line L223 (107, 66.5) -> (13, 66.5)
  line L224 (13, 66.5) -> (13, 69.5)
  line L225 (107, 39.5) -> (107, 36.5)
  line L226 (13, 39.5) -> (107, 39.5)
  line L227 (107, 36.5) -> (13, 36.5)
  line L228 (13, 36.5) -> (13, 39.5)
  line L229 (107, 49.5) -> (107, 46.5)
  line L230 (13, 49.5) -> (107, 49.5)
  line L231 (107, 46.5) -> (13, 46.5)
  line L232 (13, 46.5) -> (13, 49.5)
  line L233 (107, 59.5) -> (107, 56.5)
  line L234 (13, 59.5) -> (107, 59.5)
  line L235 (107, 56.5) -> (13, 56.5)
  line L236 (13, 56.5) -> (13, 59.5)
  line L237 (107, 39.5) -> (107, 36.5)
  line L238 (13, 39.5) -> (107, 39.5)
  line L239 (107, 36.5) -> (13, 36.5)
  line L240 (13, 36.5) -> (13, 39.5)
  line L241 (107, 49.5) -> (107, 46.5)
  line L242 (13, 49.5) -> (107, 49.5)
  line L243 (107, 46.5) -> (13, 46.5)
  line L244 (13, 46.5) -> (13, 49.5)
  line L245 (107, 39.5) -> (107, 36.5)
  line L246 (13, 39.5) -> (107, 39.5)
  line L247 (107, 36.5) -> (13, 36.5)
  line L248 (13, 36.5) -> (13, 39.5)
  line L249 (107, 29.5) -> (107, 26.5)
  line L250 (13, 29.5) -> (107, 29.5)
  line L251 (107, 26.5) -> (13, 26.5)
  line L252 (13, 26.5) -> (13, 29.5)
  line L253 (107, 39.5) -> (107, 36.5)
  line L254 (13, 39.5) -> (107, 39.5)
  line L255 (107, 36.5) -> (13, 36.5)
  line L256 (13, 36.5) -> (13, 39.5)
  line L257 (107, 49.5) -> (107, 46.5)
  line L258 (13, 49.5) -> (107, 49.5)
  line L259 (107, 46.5) -> (13, 46.5)
  line L260 (13, 46.5) -> (13, 49.5)
  line L261 (107, 59.5) -> (107, 56.5)
  line L262 (13, 59.5) -> (107, 59.5)
  line L263 (107, 56.5) -> (13, 56.5)
  line L264 (13, 56.5) -> (13, 59.5)
  line L265 (107, 29.5) -> (107, 26.5)
  line L266 (13, 29.5) -> (107, 29.5)
  line L267 (107, 26.5) -> (13, 26.5)
  line L268 (13, 26.5) -> (13, 29.5)
  line L269 (107, 39.5) -> (107, 36.5)
  line L270 (13, 39.5) -> (107, 39.5)
  line L271 (107, 36.5) -> (13, 36.5)
  line L272 (13, 36.5) -> (13, 39.5)
  line L273 (107, 49.5) -> (107, 46.5)
  line L274 (13, 49.5) -> (107, 49.5)
  line L275 (107, 46.5) -> (13, 46.5)
  line L276 (13, 46.5) -> (13, 49.5)
  line L277 (107, 29.5) -> (107, 26.5)
  line L278 (13, 29.5) -> (107, 29.5)
  line L279 (107, 26.5) -> (13, 26.5)
  line L280 (13, 26.5) -> (13, 29.5)
  line L281 (107, 39.5) -> (107, 36.5)
  line L282 (13, 39.5) -> (107, 39.5)
  line L283 (107, 36.5) -> (13, 36.5)
  line L284 (13, 36.5) -> (13, 39.5)
  line L285 (107, 29.5) -> (107, 26.5)
  line L286 (13, 29.5) -> (107, 29.5)
  line L287 (107, 26.5) -> (13, 26.5)
  line L288 (13, 26.5) -> (13, 29.5)
  point P0 (60, 0)
  point P1 (60, 76.5858)
  point P2 (13, 36.5)
  point P3 (13, 26.5)
  dimension "d59" = 119.175
  dimension "d62" = 10
  constraints: 568 end point, 3 parallel, 2 horizontal, 2 perpendicular, 1 point on line, 1 vertical, 120 other
  measures "d62" distance of L7.end L29.start
extrude "Extrusion6" cut sketch "Skizze7" against normal blind 64 contours L7 L8 L9 L10 | L13 L15 L16 L14 | L17 L19 L20 L18 | L21 L23 L24 L22 | L25 L27 L28 L26 | L29 L31 L32 L30 | L49 L51 L52 L50 | L69 L71 L72 L70 | L89 L91 L92 L90 | L109 L111 L112 L110 | L209 L211 L212 L210 | L249 L251 L252 L250
sketch "Skizze9" plane through (-60, -61, 0) normal (0, -1, 0) x (1, 0, 0)
  line L0 (120, 168) -> (0, 168) construction
  line L1 (0, 168) -> (120, 168) construction
  line L2 (120, 168) -> (120, 0) construction
  line L3 (120, 0) -> (0, 0) construction
  line L4 (0, 0) -> (0, 168) construction
  line L5 (0, 0) -> (0, 168) construction
  line L6 (120, 0) -> (120, 168) construction
  line L7 (0, 168) -> (120, 0) construction
  line L8 (120, 0) -> (120, 168) construction
  line L9 (120, 168) -> (0, 0) construction
  line L10 (2, 17) -> (118, 17)
  line L11 (118, 17) -> (118, 151)
  line L12 (118, 151) -> (2, 151)
  line L13 (2, 151) -> (2, 17)
  line L14 (2, 17) -> (118, 151) construction
  line L15 (118, 17) -> (2, 151) construction
  line L16 (111.2, 17) -> (111.2, 151)
  line L17 (8.8, 17) -> (8.8, 151)
  line L18 (109.2, 18.5) -> (109.2, 3) projected
  line L19 (10.8, 3) -> (10.8, 18.5) projected
  point P0 (60, 0)
  point P1 (60, 84)
  dimension "d67" = 116
  dimension "d68" = 134
  dimension "d69" = 2
  dimension "d70" = 2
  constraints: 30 end point, 5 equal length, 4 point on line, 3 midpoint, 3 perpendicular, 2 horizontal, 1 vertical
  measures "d67" distance of L11.end L12.end
  measures "d68" distance of L12.end L10.start
  measures "d69" distance between parallel lines of L16 L18
  measures "d70" distance between parallel lines of L17 L19
extrude "Extrusion7" cut sketch "Skizze9" against normal blind 112 contours L13 L12 L17 L10 | L12 L11 L10 L16
sketch "Skizze10" plane through (0, 0, 168) normal (0, 0, 1) x (1, 0, 0)
  line L0 (-60, -61) -> (-45.2253, -75.7747)
  line L1 (60, -61) -> (38.3771, -82.6229)
  line L2 (45, -61) -> (60, -61) projected
  line L3 (49.2, -61) -> (57.6103, -69.4103)
  line L4 (-60, -61) -> (-45, -61) projected
  line L5 (-49.2, -61) -> (-65.8786, -77.6786)
  line L6 (-58, -61) -> (-58, 51) projected
  line L7 (-58, -61) -> (-51.9282, -67.0718)
  line L8 (-51.2, -61) -> (-58.5393, -68.3393)
  line L9 (51.2, -61) -> (51.2, 51) projected
  line L10 (51.2, -61) -> (57.955, -67.755)
  line L11 (58, -61) -> (58, 51) projected
  line L12 (57.955, -67.755) -> (58, -61)
  line L13 (58, -61) -> (52.5, -66.5)
  point P0 (0, 0)
  point P1 (54.6, -64.4)
  point P2 (54.6, -66.4)
  point P3 (57.9866, -63.0134)
  point P4 (-54.6, -64.4)
  point P5 (-54.6, -66.4)
  dimension "d73" = 45
  dimension "d74" = 45
  dimension "d75" = 45
  dimension "d76" = 45
  dimension "d77" = 2
  dimension "d78" = 2
  constraints: 18 end point, 2 parallel, 2 point on line, 1 perpendicular
  measures "d73" angle of L4 L5
  measures "d74" angle of L4 L0
  measures "d75" angle of L2 L3
  measures "d76" angle of L2 L1
  measures "d77" distance of L3.start L9.start
  measures "d78" distance of L5.start L8.start
extrude "Extrusion8" add sketch "Skizze10" against normal up to surface (168 mm away) contours L4 L7 L8 L0 | L8 L7 L5 L0 | L8 L4 L5 L7 | L1 L12 L2 | L1 L10 L13 L12 | L1 L3 L13 L10 | L10 L13 L3 L2
sketch "Skizze11" plane through (0, 0, 168) normal (0, 0, 1) x (1, 0, 0)
  line L0 (-51.2, -61) -> (-58, -61) projected
  line L1 (-51.2, -61) -> (-54.6, -64.4) projected
  line L2 (-58, -61) -> (-51.2, -61)
  line L3 (-51.2, -61) -> (-54.6, -64.4)
  line L4 (-58, -61) -> (-54.6, -64.4) projected
  line L5 (-54.6, -64.4) -> (-58, -61)
  line L6 (51.2, -61) -> (58, -61) projected
  line L7 (54.6, -64.4) -> (51.2, -61) projected
  line L8 (51.2, -61) -> (54.6, -64.4)
  line L9 (54.6, -64.4) -> (58, -61)
  line L10 (58, -61) -> (51.2, -61)
  point P0 (0, 0)
  constraints: 12 end point, 3 collinear, 2 horizontal, 1 perpendicular
extrude "Extrusion9" add sketch "Skizze11" against normal blind 2
sketch "Skizze12" plane through (0, 0, 0) normal (0, 0, -1) x (-1, 0, 0)
  line L0 (58, -61) -> (54.6, -64.4) projected
  line L1 (54.6, -64.4) -> (51.2, -61)
  line L2 (51.2, -61) -> (58, -61) projected
  line L3 (51.2, -61) -> (58, -61)
  line L4 (58, -61) -> (54.6, -64.4)
  line L5 (-51.2, -61) -> (-58, -61) projected
  line L6 (-51.2, -61) -> (-58, -61)
  line L7 (-54.6, -64.4) -> (-58, -61) projected
  line L8 (-58, -61) -> (-54.6, -64.4)
  line L9 (-54.6, -64.4) -> (-51.2, -61)
  point P0 (0, 0)
  constraints: 12 end point, 3 collinear, 3 perpendicular
extrude "Extrusion10" add sketch "Skizze12" against normal blind 2
sketch "Skizze13" plane through (0, 0, 0) normal (0, 0, -1) x (-1, 0, 0)
  line L0 (-60, 61) -> (60, 61) construction
  line L1 (-60, -61) -> (-60, 61) construction
  line L2 (60, 61) -> (-60, 61) construction
  line L3 (-60, 61) -> (-60, -61) construction
  line L4 (-60, -61) -> (60, -61) construction
  line L5 (60, -61) -> (60, 61) construction
  line L6 (60, 61) -> (60, -61) construction
  line L7 (60, -61) -> (-60, 61) construction
  line L8 (-60, -61) -> (60, 61) construction
  line L9 (60, -46) -> (-60, -46) construction
  line L10 (60, 46) -> (-60, 46) construction
  line L11 (49.2, -61) -> (45, -61) construction
  line L12 (60, -46) -> (45, -61) construction
  line L13 (-45, -59) -> (-45, -61) construction
  line L14 (-60, -46) -> (-45, -61) construction
  line L15 (-60, 46) -> (-45, 61) construction
  line L16 (44.8371, 45.75) -> (44.8371, 61) construction
  line L17 (60, 46) -> (45, 61) construction
  line L18 (47.5, -58.5) -> (57.5, -58.5)
  line L19 (57.5, -58.5) -> (57.5, -48.5)
  line L20 (57.5, -48.5) -> (47.5, -48.5)
  line L21 (47.5, -48.5) -> (47.5, -58.5)
  line L22 (47.5, -58.5) -> (57.5, -48.5) construction
  line L23 (57.5, -58.5) -> (47.5, -48.5) construction
  line L24 (-47.5, -58.5) -> (-57.5, -58.5)
  line L25 (-57.5, -58.5) -> (-57.5, -48.5)
  line L26 (-57.5, -48.5) -> (-47.5, -48.5)
  line L27 (-47.5, -48.5) -> (-47.5, -58.5)
  line L28 (-47.5, -58.5) -> (-57.5, -48.5) construction
  line L29 (-57.5, -58.5) -> (-47.5, -48.5) construction
  line L30 (-47.5, 48.5417) -> (-57.5, 48.5417)
  line L31 (-57.5, 48.5417) -> (-57.5, 58.4583)
  line L32 (-57.5, 58.4583) -> (-47.5, 58.4583)
  line L33 (-47.5, 58.4583) -> (-47.5, 48.5417)
  line L34 (-47.5, 48.5417) -> (-57.5, 58.4583) construction
  line L35 (-57.5, 48.5417) -> (-47.5, 58.4583) construction
  line L36 (57.4583, 48.5417) -> (47.5417, 48.5417)
  line L37 (47.5417, 48.5417) -> (47.5417, 58.4583)
  line L38 (47.5417, 58.4583) -> (57.4583, 58.4583)
  line L39 (57.4583, 58.4583) -> (57.4583, 48.5417)
  line L40 (57.4583, 48.5417) -> (47.5417, 58.4583) construction
  line L41 (47.5417, 48.5417) -> (57.4583, 58.4583) construction
  point P0 (0, 0)
  point P1 (52.5, -53.5)
  point P2 (-52.5, -53.5)
  point P3 (-52.5, 53.5)
  point P4 (52.5, 53.5)
  dimension "d25" = 10
  dimension "d28" = 10
  dimension "d85" = 15
  dimension "d86" = 15
  dimension "d87" = 10
  dimension "d98" = 10
  constraints: 72 end point, 12 midpoint, 12 point on line, 11 parallel, 6 horizontal, 6 perpendicular
  measures "d85" distance between parallel lines of L0 L10
  measures "d86" distance between parallel lines of L9 L4
  measures "d87" distance of L18.start L18.end
  measures "d98" distance of L18.end L19.end
extrude "Extrusion11" cut sketch "Skizze13" against normal blind 3
sketch "Skizze14" plane through (0, 0, 0) normal (0, 0, -1) x (-1, 0, 0)
  line L0 (45, -59) -> (47, -59) projected
  line L1 (45, 3) -> (45, -43.5) projected
  line L2 (47, -59) -> (45, -59)
  line L3 (45, -59) -> (45, -43.5)
  line L4 (45, -43.5) -> (47, -43.5)
  line L5 (47, -43.5) -> (47, -59)
  line L6 (-45, -59) -> (-47, -59) projected
  line L7 (-47, -43.5) -> (-45, -43.5) projected
  line L8 (-45, -59) -> (-47, -59)
  line L9 (-47, -59) -> (-47, -43.5)
  line L10 (-47, -43.5) -> (-45, -43.5)
  line L11 (-45, -43.5) -> (-45, -59)
  point P0 (0, 0)
  point P1 (-47, -59)
  constraints: 16 end point, 4 parallel, 2 horizontal, 2 perpendicular
extrude "Extrusion12" add sketch "Skizze14" against normal blind 3
sketch "Skizze15" plane through (45, -61, 159.5) normal (0, -1, 0) x (1, 0, 0)
  line L0 (4.2, -141) -> (4.2, -156.5) projected
  line L1 (-94.2, -156.5) -> (-94.2, -141) projected
  point P0 (-45, -159.5)
  dimension "d92" = 98.4
  measures "d92" distance between parallel lines of L0 L1
sketch "Skizze17" plane through (-45, -61, 159.5) normal (0, -1, 0) x (1, 0, 0)
  line L0 (92, -20) -> (92, -23) projected
  line L1 (-2, -13) -> (-2, -10) projected
  line L2 (90, -70) -> (92, -70) projected
  line L3 (92, -73) -> (90, -73) projected
  point P0 (45, -159.5)
  point P1 (92, -80)
  point P2 (92, -83)
  point P3 (-2, -83)
  point P4 (-2, -80)
  dimension "d94" = 94
  dimension "d95" = 3
  measures "d94" distance between parallel lines of L0 L1
  measures "d95" distance between parallel lines of L2 L3
sketch "Skizze18" plane through (0, 0, 168) normal (0, 0, 1) x (1, 0, 0)
  line L0 (-60, 61) -> (-60, -61) construction
  line L1 (60, -61) -> (60, 61) construction
  line L2 (-60, -61) -> (60, 61) construction
  line L3 (60, 61) -> (-60, 61) construction
  line L4 (-58, 51) -> (-51.2, 51) construction
  line L5 (-60, 61) -> (60, -61) construction
  line L6 (60, -61) -> (-60, -61) construction
  line L7 (-58, -61) -> (-58, 51) construction
  point P0 (0, 0)
  dimension "d97" = 61
  constraints: 8 end point, 1 parallel, 1 perpendicular
  measures "d97" distance from line of L6 point (0, 0)
sketch "Skizze19" plane through (0, 0, 168) normal (0, 0, 1) x (1, 0, 0)
  line L0 (60, -61) -> (60, 61) projected
  line L1 (45, 45.75) -> (45, -43.5) projected
  point P0 (0, 0)
  dimension "d99" = 15
  measures "d99" distance between parallel lines of L0 L1
sketch "Skizze20" plane through (0, 0, 168) normal (0, 0, 1) x (1, 0, 0)
  line L0 (-60, 61) -> (-60, -61) projected
  line L1 (44.9854, 61) -> (44.9854, 45.75) projected
  line L2 (-60, 61) -> (44.9854, 61)
  line L3 (44.9854, 61) -> (44.9854, 45.75)
  line L4 (44.9854, 45.75) -> (-60, 45.75)
  line L5 (-60, 45.75) -> (-60, 61)
  line L6 (60, -61) -> (60, 61) projected
  line L7 (44.9854, 61) -> (60, 61)
  line L8 (60, 61) -> (60, 45.75)
  line L9 (60, 45.75) -> (44.9854, 45.75)
  line L10 (44.9854, 45.75) -> (44.9854, 61)
  line L11 (-60, -60.989) -> (60, -60.989)
  line L12 (60, -60.989) -> (60, -66.7212)
  line L13 (60, -66.7212) -> (-60, -66.7212)
  line L14 (-60, -66.7212) -> (-60, -60.989)
  point P0 (0, 0)
  point P1 (-45, 61)
  constraints: 24 end point, 6 parallel, 4 point on line, 3 horizontal, 3 perpendicular
extrude "Extrusion13" cut sketch "Skizze20" against normal up to surface (168 mm away) contours L2 L1 L4 L0 | L7 L6 L9 L1 | L11 L6 L12 L13 L14 L0
sketch "Skizze21" plane through (-60, -60.989, 168) normal (0, -1, 0) x (1, 0, 0)
  line L0 (2, -17) -> (2, -151) projected
  line L1 (2.5, -136) -> (8.8, -136) projected
  line L2 (2, -17) -> (8.8, -17)
  line L3 (8.8, -17) -> (8.8, -136)
  line L4 (8.8, -136) -> (2, -136)
  line L5 (2, -136) -> (2, -17)
  line L6 (111.2, -17) -> (111.2, -151) projected
  line L7 (118, -17) -> (118, -151) projected
  line L8 (111.2, -17) -> (118, -17)
  line L9 (118, -17) -> (118, -151)
  line L10 (118, -151) -> (111.2, -151)
  line L11 (111.2, -151) -> (111.2, -17)
  line L12 (2, -151) -> (8.8, -151) projected
  line L13 (2, -136) -> (2, -151)
  line L14 (2, -151) -> (8.8, -151)
  line L15 (8.8, -151) -> (8.8, -136)
  point P0 (60, -168)
  point P1 (2, -136)
  constraints: 22 end point, 5 equal length, 3 perpendicular, 2 horizontal, 1 vertical
extrude "Extrusion14" add sketch "Skizze21" against normal up to surface (106.739 mm away)